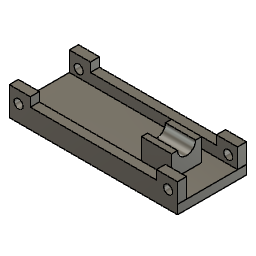
logo_sides (Autodesk Fusion 360 design; units mm, degrees)
Autodesk Fusion 360 part; units mm, degrees
note: some values were not read from the file. Set by a fixed rule: which sketch regions a step uses.
sketch "Sketch1" plane through (0, 0, 0) normal (0, 1, 0) x (1, 0, 0)
  line L0 (0, 0) -> (56, 0)
  line L1 (56, 0) -> (56, -23)
  line L2 (56, -23) -> (0, -23)
  line L3 (0, -23) -> (0, 0)
  dimension "d1" = 56
  dimension "d2" = 23
  constraint horizontal L0
  constraint vertical L1
  constraint horizontal L2
  constraint vertical L3
  constraint coincident L0.start L3.end
  measures "d1" distance of L0.start L0.end
  measures "d2" distance of L0.start L2.end
extrude "Extrude1" add sketch "Sketch1" along normal blind 3
sketch "Sketch2" plane through (0, 3, 0) normal (0, 1, 0) x (-1, 0, 0)
  line L0 (0, 23) -> (-56, 23)
  line L1 (-56, 23) -> (-56, 0)
  line L2 (-56, 0) -> (0, 0)
  line L3 (0, 0) -> (0, 23)
  line L4 (0, 0) -> (-55.9429, 0)
  line L5 (-55.9429, 0) -> (-55.9429, 7.5)
  line L6 (-55.9429, 7.5) -> (0, 7.5)
  line L7 (0, 7.5) -> (0, 0)
  line L8 (0, 11.5) -> (-56, 11.5)
  line L9 (-55.9429, 15.5) -> (0, 15.5)
  line L10 (0, 15.5) -> (0, 23)
  line L11 (0, 23) -> (-56, 23)
  line L12 (-55.9429, 15.5) -> (-56, 23)
  line L13 (0, 7.5) -> (-7.5, 7.5)
  line L14 (-7.5, 7.5) -> (-7.5, 4.5)
  line L15 (-55.9429, 7.5) -> (-48.4429, 7.5)
  line L16 (-48.4429, 7.5) -> (-48.4429, 4.5)
  line L17 (-7.5, 4.5) -> (-48.4429, 4.5)
  line L18 (-48.4429, 4.5) -> (-48.4429, 7.5)
  line L19 (-7.5, 18.5) -> (-48.4429, 18.5)
  line L20 (-48.4429, 15.5) -> (-48.4429, 18.5)
  line L21 (-7.5, 15.5) -> (-7.5, 18.5)
  line L22 (0, 0) -> (0, 3)
  line L23 (0, 3) -> (-56, 3)
  line L24 (0, 20) -> (-56, 20)
  dimension "d5" = 7.5
  dimension "d6" = 7.5
  dimension "d7" = 3
  dimension "d8" = 7.5
  dimension "d9" = 3
  dimension "d10" = 3
  constraint horizontal L4
  constraint vertical L5
  constraint horizontal L6
  constraint vertical L7
  constraint coincident L2.end L3.start
  constraint midpoint L3 L8.start
  constraint midpoint L1 L8.end
  constraint symmetric L5.end L8 L9.start
  constraint symmetric L6.end L8 L9.end
  constraint coincident L0.start L3.end
  constraint coincident L0.end L1.start
  constraint perpendicular L3 L13
  constraint perpendicular L13 L14
  constraint perpendicular L1 L15
  constraint perpendicular L15 L16
  constraint symmetric L8 L13.end L21.start
  constraint symmetric L8 L14.end L19.start
  constraint symmetric L8 L15.end L20.start
  constraint symmetric L8 L16.end L19.end
  constraint perpendicular L2 L22
  constraint coincident L1 L23.end
  constraint perpendicular L1 L23
  constraint symmetric L8 L22.end L24.start
  constraint symmetric L8 L23.end L24.end
  measures "d5" distance of L2.end L6.end
  measures "d6" distance of L6.end L13.end
  measures "d7" distance of L13.end L14.end
  measures "d8" distance of L5.end L15.end
  measures "d9" distance of L15.end L16.end
  measures "d10" distance of L2.end L22.end
extrude "Extrude2" add sketch "Sketch2" along normal blind 6.5 contours L0 L3 L10 L11 L12 L24 | L2 L3 L4 L5 L7 L22 L23
sketch "Sketch3" plane through (0, 0, 0) normal (0, 0, -1) x (-1, 0, 0)
  line L0 (-56, 0) -> (0, 0)
  line L1 (0, 0) -> (0, 9.5)
  line L2 (0, 9.5) -> (-55.9429, 9.5)
  line L3 (-55.9429, 9.5) -> (-55.9429, 3)
  line L4 (-55.9429, 3) -> (-56, 3)
  line L5 (-56, 3) -> (-56, 0)
  line L6 (0, 0) -> (0, 9.5)
  line L7 (0, 9.5) -> (-7, 9.5)
  line L8 (-7, 9.5) -> (-7, 6.5)
  line L9 (-55.9429, 9.5) -> (-48.9429, 9.5)
  line L10 (-48.9429, 9.5) -> (-48.9429, 6.5)
  line L11 (-7, 6.5) -> (-48.9429, 6.5)
  dimension "d13" = 9.5
  dimension "d14" = 7
  dimension "d15" = 3
  dimension "d16" = 7
  dimension "d17" = 3
  constraint coincident L0.end L1.start
  constraint coincident L1.end L2.start
  constraint perpendicular L1 L7
  constraint perpendicular L2 L8
  constraint coincident L2.end L3.start
  constraint perpendicular L3 L9
  constraint perpendicular L2 L10
  measures "d13" distance of L0.end L1.end
  measures "d14" distance of L1.end L7.end
  measures "d15" distance of L7.end L8.end
  measures "d16" distance of L2.end L9.end
  measures "d17" distance of L9.end L10.end
extrude "Extrude3" cut sketch "Sketch3" against normal blind 30 contours L2 L8 L10 L11
sketch "Sketch4" plane through (0, 0, 0) normal (0, 0, -1) x (-1, 0, 0)
  line L0 (-7, 9.5) -> (-7, 6.5)
  line L1 (-7, 6.5) -> (-48.9429, 6.5)
  line L2 (-48.9429, 6.5) -> (-48.9429, 9.5)
  line L3 (-48.9429, 9.5) -> (-55.9429, 9.5)
  line L4 (-55.9429, 9.5) -> (-55.9429, 3)
  line L5 (-55.9429, 3) -> (-56, 3)
  line L6 (-56, 3) -> (-56, 0)
  line L7 (-56, 0) -> (0, 0)
  line L8 (0, 0) -> (0, 9.5)
  line L9 (0, 9.5) -> (-7, 9.5)
  line L10 (0, 0) -> (-3.081, 0)
  line L11 (-3.081, 0) -> (-3.081, 9.5)
  line L12 (0, 0) -> (0, 2.916)
  line L13 (0, 2.916) -> (-5.2666, 2.916)
  line L14 (-28, 0) -> (-27.9715, 6.5)
  line L15 (-2.393, 9.5) -> (-2.393, 6.584)
  line L16 (-2.393, 6.584) -> (-5.7836, 6.584)
  line L17 (-3.081, 0) -> (-3.081, 4.5)
  line L18 (-3.081, 0) -> (-3.081, 5.5)
  circle A0 centre (-3.081, 5.5) radius 1.5
  circle A1 centre (-52.8697, 5.7187) radius 1.5
  dimension "d20" = 3.081
  dimension "d21" = 2.916
  dimension "d23" = 2.916
  dimension "d25" = 4.5
  dimension "d26" = 5.5
  dimension "d27" = 3
  constraint coincident L7.end L8.start
  constraint perpendicular L8 L10
  constraint coincident L9 L11.end
  constraint perpendicular L9 L11
  constraint perpendicular L7 L12
  constraint perpendicular L11 L13
  constraint midpoint L7 L14.start
  constraint midpoint L1 L14.end
  constraint coincident L9 L15.start
  constraint perpendicular L9 L15
  constraint perpendicular L0 L16
  constraint perpendicular L7 L17
  constraint perpendicular L7 L18
  constraint coincident L18.end A0.centre
  constraint symmetric L14 A0 A1
  measures "d20" distance of L7.end L10.end
  measures "d21" distance of L7.end L12.end
  measures "d23" distance of L15.start L15.end
  measures "d25" distance of L10.end L17.end
  measures "d26" distance of L10.end L18.end
  measures "d27" diameter of A0
extrude "Extrude4" cut sketch "Sketch4" against normal blind 30 contours L11 L15 L16 A0 | L11 L16 A0 | L11 L15 L16 L17 L18 A0 | L11 L16 L17 L18 A0 | A1
sketch "Sketch6" plane through (0, 3, 0) normal (0, 1, 0) x (-1, 0, 0)
  line L0 (-55.9772, 20) -> (-56, 23)
  line L1 (-56, 23) -> (-56, 0)
  line L2 (-56, 0) -> (-55.9429, 0)
  line L3 (-55.9429, 0) -> (-55.9429, 3)
  line L4 (-55.9429, 3) -> (0, 3)
  line L5 (0, 3) -> (0, 20)
  line L6 (0, 20) -> (-55.9772, 20)
  line L7 (-55.9772, 20) -> (-47.9772, 20)
  line L8 (-47.9772, 20) -> (-37.9772, 20)
  line L9 (-37.9772, 20) -> (-37.9772, 10)
  line L10 (-37.9772, 10) -> (-47.9772, 10)
  line L11 (-47.9772, 10) -> (-47.9772, 20)
  line L12 (-37.9772, 20) -> (-37.9772, 19.4199)
  line L13 (-37.9772, 3) -> (-37.9772, 20)
  line L14 (-37.9772, 20) -> (-37.9772, 11.5)
  line L15 (-37.9772, 17) -> (-37.9772, 8.5)
  line L16 (-37.9772, 17) -> (-37.9772, 7)
  line L17 (-37.9772, 7) -> (-47.9772, 7)
  line L18 (-47.9772, 7) -> (-47.9772, 17)
  line L19 (-47.9772, 17) -> (-37.9772, 17)
  dimension "d30" = 8
  dimension "d31" = 10
  dimension "d32" = 10
  dimension "d38" = 10
  dimension "d39" = 10
  constraint coincident L0.start L6.end
  constraint perpendicular L1 L7
  constraint horizontal L8
  constraint vertical L9
  constraint horizontal L10
  constraint vertical L11
  constraint coincident L9 L12.end
  constraint perpendicular L6 L12
  constraint coincident L4 L13.start
  constraint perpendicular L6 L13
  constraint midpoint L13 L14.end
  constraint horizontal L19
  constraint vertical L16
  constraint horizontal L17
  constraint vertical L18
  measures "d30" distance of L0.start L7.end
  measures "d31" distance of L7.end L8.end
  measures "d32" distance of L7.end L10.end
  measures "d38" distance of L15.start L18.end
  measures "d39" distance of L17.end L18.end
extrude "Extrude5" add sketch "Sketch6" along normal blind 7.5 contours L9 L10 L11 L13 L14 L15 L16 L18 L19 | L10 L13 L15 L16 L17 L18
sketch "Sketch7" plane through (47.9772, 0, 0) normal (1, 0, 0) x (0, 0, -1)
  line L0 (-17, 3) -> (-7, 3)
  line L1 (-7, 10.5) -> (-17, 10.5)
  circle A0 centre (-12, 10.5) radius 3
  line L2 (-7, 3) -> (-7, 10.5)
  line L3 (-17, 10.5) -> (-17, 3)
  dimension "d35" = 6
  constraint midpoint L1 A0.centre
  measures "d35" diameter of A0
extrude "Extrude6" cut sketch "Sketch7" against normal blind 10 contours L1 A0 picked at (-12.5, 9.634)
